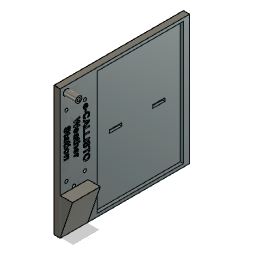
SolarPanelHolder (Autodesk Fusion 360 design; units mm, degrees)
Autodesk Fusion 360 part; units mm, degrees
sketch "Sketch1" plane through (0, 0, 0) normal (1, 0, 0) x (0, 0, -1)
  line L0 (0, -105) -> (80, -105)
  line L1 (0, -105) -> (-95, -105)
  line L2 (0, 105) -> (80, 105)
  line L3 (80, 105) -> (80, -105)
  line L4 (80, 105) -> (80, 100)
  line L5 (80, 100) -> (70, 100)
  line L6 (-95, 105) -> (-130, 105)
  line L7 (-95, 105) -> (0, 105)
  line L8 (-130, 105) -> (-130, -105)
  line L9 (-130, -105) -> (-95, -105)
  dimension "d1" = 105
  dimension "d2" = 105
  dimension "d3" = 80
  dimension "d4" = 95
  dimension "d5" = 95
  dimension "d6" = 80
  dimension "d7" = 5
  dimension "d8" = 10
  dimension "d9" = 35
  constraint perpendicular L2 L4
  constraint perpendicular L4 L5
  constraint parallel L2 L7
  constraint perpendicular L6 L8
  constraint perpendicular L8 L9
  measures "d1" distance of origin L2.start
  measures "d2" distance of origin L0.start
  measures "d3" distance of L0.start L0.end
  measures "d4" distance of L0.start L1.end
  measures "d5" distance of L2.start L6.start
  measures "d6" distance of L2.start L2.end
  measures "d7" distance of L2.end L4.end
  measures "d8" distance of L4.end L5.end
  measures "d9" distance of L6.start L6.end
extrude "Extrude1" add sketch "Sketch1" along normal blind 5
sketch "Sketch2" plane through (5, 0, 0) normal (1, 0, 0) x (0, 0, -1)
  line L0 (80, 105) -> (-130, 105)
  line L1 (-130, 105) -> (-130, -105)
  line L2 (-130, -105) -> (80, -105)
  line L3 (80, -105) -> (80, 105)
  line L4 (80, 105) -> (80, 100)
  line L5 (80, 100) -> (70, 100)
  line L6 (70, 100) -> (70, -100)
  line L7 (70, -100) -> (-70, -100)
  line L8 (-70, -100) -> (-70, 100)
  line L9 (-70, 100) -> (70, 100)
  dimension "d12" = 5
  dimension "d13" = 10
  constraint coincident L0.start L3.end
  constraint perpendicular L0 L4
  constraint perpendicular L4 L5
  constraint perpendicular L5 L6
  constraint perpendicular L6 L7
  constraint perpendicular L7 L8
  constraint perpendicular L6 L9
  measures "d12" distance of L0.start L4.end
  measures "d13" distance of L4.end L5.end
extrude "Extrude2" add sketch "Sketch2" along normal blind 5
sketch "Sketch3" plane through (10, 0, 0) normal (1, 0, 0) x (0, 0, -1)
  line L0 (-70, -100) -> (-70, 100)
  line L1 (-70, 100) -> (70, 100)
  line L2 (70, 100) -> (70, -100)
  line L3 (70, -100) -> (-70, -100)
  line L4 (-130, 105) -> (-130, -105)
  line L5 (-130, -105) -> (80, -105)
  line L6 (80, -105) -> (80, 105)
  line L7 (80, 105) -> (-130, 105)
sketch "Sketch4" plane through (0, 0, 130) normal (0, 0, 1) x (1, 0, 0)
  line L0 (0, 105) -> (0, -105)
  line L1 (0, -105) -> (10, -105)
  line L2 (10, -105) -> (10, 105)
  line L3 (10, 105) -> (0, 105)
  line L4 (10, -105) -> (10, -45)
  line L5 (10, -45) -> (30, -45)
  line L6 (30, -45) -> (10, -105)
  dimension "d19" = 60
  dimension "d20" = 20
  constraint coincident L1.end L2.start
  constraint perpendicular L1 L4
  constraint perpendicular L2 L5
  measures "d19" distance of L1.end L4.end
  measures "d20" distance of L4.end L5.end
extrude "Extrude3" add sketch "Sketch4" against normal blind 45 contours L2 L4 L5 L6
sketch "Sketch5" plane through (10, 0, 0) normal (1, 0, 0) x (0, 0, -1)
  circle A0 centre (-120, 95) radius 5
  dimension "d24" = 10
  measures "d24" diameter of A0
extrude "Extrude4" add sketch "Sketch5" along normal blind 20
sketch "Sketch6" plane through (30, 0, 0) normal (1, 0, 0) x (0, 0, -1)
  circle A0 centre (-120, 95) radius 5
  circle A1 centre (-120, 95) radius 2.5
  dimension "d27" = 5
  constraint concentric A0 A1
  measures "d27" diameter of A1
extrude "Extrude5" cut sketch "Sketch6" against normal blind 50 contours A1
sketch "Sketch7" plane through (10, 0, 0) normal (1, 0, 0) x (0, 0, -1)
  circle A0 centre (-107.6033, -42.5318) radius 2.5
  dimension "d30" = 5
  measures "d30" diameter of A0
extrude "Extrude6" cut sketch "Sketch7" against normal blind 70
sketch "Sketch8" plane through (10, 0, 0) normal (1, 0, 0) x (0, 0, -1)
  line L0 (25, 0) -> (25, -2.5)
  line L1 (25, 0) -> (25, 2.5)
  line L2 (25, 2.5) -> (45, 2.5)
  line L3 (25, -2.5) -> (45, -2.5)
  line L4 (45, -2.5) -> (45, 2.5)
  line L5 (-45, 0) -> (-45, 2.5)
  line L6 (-45, 0) -> (-45, -2.5)
  line L7 (-25, 0) -> (-25, 2.5)
  line L8 (-25, 0) -> (-25, -2.5)
  line L9 (-45, 2.5) -> (-25, 2.5)
  line L10 (-45, -2.5) -> (-25, -2.5)
  dimension "d36" = 2.5
  dimension "d37" = 2.5
  dimension "d38" = 20
  dimension "d39" = 20
  dimension "d43" = 2.5
  dimension "d44" = 2.5
  dimension "d45" = 2.5
  dimension "d46" = 2.5
  constraint perpendicular L1 L2
  constraint perpendicular L0 L3
  constraint perpendicular L2 L4
  measures "d36" distance of L0.start L0.end
  measures "d37" distance of L0.start L1.end
  measures "d38" distance of L1.end L2.end
  measures "d39" distance of L0.end L3.end
  measures "d43" distance of L5.start L5.end
  measures "d44" distance of L5.start L6.end
  measures "d45" distance of L7.start L7.end
  measures "d46" distance of L7.start L8.end
extrude "Extrude7" cut sketch "Sketch8" against normal blind 9
sketch "Sketch9" plane through (10, 0, 0) normal (1, 0, 0) x (0, 0, -1)
  line L0 (-128.3815, 78.5203) -> (-128.0373, -32.6148) construction
  line L1 (-128.0373, -32.6148) -> (-82.099, -32.4725) construction
  line L2 (-82.099, -32.4725) -> (-82.4432, 78.6625) construction
  line L3 (-82.4432, 78.6625) -> (-128.3815, 78.5203) construction
  dimension "d49" = 10
  text T0 "e-CALLISTO\nWeather\nStation" font "Arial" height 10 bold align centre top in box 111.1356 x 45.9385 at (-128.3815, 78.5203) x (0.003097, -0.999995) y (0.999995, 0.003097) spacing 1 kerned
extrude "Extrude8" cut sketch "Sketch9" against normal blind 5 text T0
sketch "Sketch10" plane through (10, 0, 0) normal (1, 0, 0) x (0, 0, -1)
  circle A0 centre (-120, 70) radius 2.5
  circle A1 centre (-90, 70) radius 2.5
  circle A2 centre (-120, -30) radius 2.5
  circle A3 centre (-90, -30) radius 2.5
  dimension "d52" = 5
  dimension "d53" = 5
  dimension "d54" = 5
  dimension "d55" = 5
  measures "d52" diameter of A0
  measures "d53" diameter of A1
  measures "d54" diameter of A2
  measures "d55" diameter of A3
extrude "Extrude9" cut sketch "Sketch10" against normal blind 20
